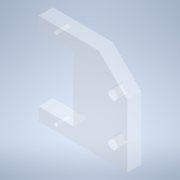
# Autodesk Inventor part: Adaptador SG90
Saved by Autodesk Inventor 2020.3 (Build 243373000, 373)
## iProperties
Created: 2021-02-24
Part Number: Adaptador SG90
Material: PET Plastic
Document SubType Name: Modeling
Designer: juanp
Density: 1.541 g/cm^3
Appearance: Polycarbonate - Clear
Mass: 3.4579 g
Surface Area: 22.6075 cm^2
Volume: 3.4579 cm^3
Author: juanp
Autodesk Inventor part; units mm, degrees
ref_plane "YZ Plane" through (0, 0, 0) normal (1, 0, 0) x (0, 1, 0)
ref_plane "XZ Plane" through (0, 0, 0) normal (0, 1, 0) x (-1, 0, 0)
ref_plane "XY Plane" through (0, 0, 0) normal (0, 0, 1) x (1, 0, 0)
sketch "Sketch1" plane through (0, 0, 0) normal (0, 0, 1) x (1, 0, 0)
  line L0 (0, 0) -> (0, 4.8)
  line L1 (0, 4.8) -> (31.1, 4.8)
  line L2 (31.1, 4.8) -> (31.1, -27.3)
  line L3 (31.1, -27.3) -> (0, -27.3)
  line L4 (0, -27.3) -> (0, -22.5)
  line L5 (0, -22.5) -> (12.2, -22.5)
  line L6 (12.2, -22.5) -> (12.2, 0)
  line L7 (12.2, 0) -> (0, 0)
  line L8 (6.1, 0) -> (6.1, 2.65) construction
  line L9 (6.1, 2.65) -> (6.1, 4.8) construction
  line L10 (12.2, -11.25) -> (7.9723, -11.25) construction
  circle A0 centre (6.1, 2.65) radius 0.625
  line L11 (6.1, -22.5) -> (6.1, -25.15) construction
  line L12 (6.1, -25.15) -> (6.1, -27.3) construction
  circle A1 centre (6.1, -25.15) radius 0.625
  line L13 (26.1, -27.3) -> (26.1, -21.25) construction
  line L14 (26.1, -21.25) -> (26.1, -6.25) construction
  circle A2 centre (26.1, -6.25) radius 1.65
  circle A3 centre (26.1, -21.25) radius 1.65
  line L15 (0, 0) -> (12.2, 0)
  line L16 (12.2, 0) -> (12.2, 0.25)
  line L17 (12.2, 0.25) -> (0, 0.25)
  line L18 (0, 0.25) -> (0, 0)
  line L19 (0, -22.5) -> (12.2, -22.5)
  line L20 (12.2, -22.5) -> (12.2, -22.75)
  line L21 (12.2, -22.75) -> (0, -22.75)
  line L22 (0, -22.75) -> (0, -22.5)
  point P0 (0, -22.75)
  dimension "d0" = 22.5
  dimension "d1" = 12.2
  dimension "d2" = 4.8
  dimension "d3" = 18.9
  dimension "d4" = 2.15
  dimension "d5" = 1.25
  dimension "d10" = 5
  dimension "d11" = 3.3
  dimension "d12" = 15
  dimension "d13" = 6.05
  dimension "d17" = 0.25
  dimension "d18" = 0.25
  constraints: 46 end point, 8 perpendicular, 8 point on line, 4 centre point, 4 coincident, 4 parallel, 4 symmetric about line, 3 horizontal, 3 vertical, 2 collinear, 2 midpoint, 1 equal radius, 1 other
  measures "d0" distance between parallel lines of L7 L5
  measures "d1" distance between parallel lines of L0 L6
  measures "d2" distance between parallel lines of L5 L3
  measures "d3" distance between parallel lines of L6 L2
  measures "d4" distance of L8.end L9.end
  measures "d5" diameter of A0
  measures "d10" distance between parallel lines of L13 L2
  measures "d11" diameter of A2
  measures "d12" distance of L13.end L14.end
  measures "d13" distance of L13.start L13.end
  measures "d17" distance between parallel lines of L17 L7
  measures "d18" distance between parallel lines of L5 L21
extrude "Extrusion1" add sketch "Sketch1" along normal blind 5 contours L0 L1 L2 L3 L4 L21 L20 L6 L16 L17
chamfer "Chamfer1" distance 10 angle 45 1 edges at (31.1, 4.8, 2.5)
body "Solid1"
